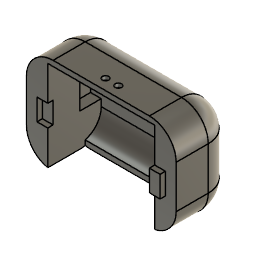
part - head front (Autodesk Fusion 360 design; units mm, degrees)
Autodesk Fusion 360 part; units mm, degrees
note: some values were not read from the file. Set by a fixed rule: which sketch regions a step uses.
sketch "Sketch6" plane through (0, 0, 0) normal (1, 0, 0) x (0, 1, 0)
  line L0 (30, 45) -> (-30, 45)
  line L1 (-55, 20) -> (-55, -20)
  line L2 (-30, -45) -> (30, -45)
  line L3 (55, -20) -> (55, 20)
  line L4 (55, 45) -> (-55, -45) construction
  line L5 (-55, 45) -> (55, -45) construction
  arc A0 (-55, -20) -> (-30, -45) centre (-30, -20) ccw
  arc A1 (55, 20) -> (30, 45) centre (30, 20) ccw
  arc A2 (-30, 45) -> (-55, 20) centre (-30, 20) ccw
  arc A3 (30, -45) -> (55, -20) centre (30, -20) ccw
  dimension "d55" = 110
  dimension "d56" = 90
  dimension "d57" = 25
  constraint horizontal L0
  constraint perpendicular L0 L1
  constraint parallel L0 L2
  constraint parallel L1 L3
  constraint coincident L4 origin
  constraint coincident L5 origin
  constraint coincident L4.end L1
  constraint coincident L4.end L2
  constraint tangent L1 A0
  constraint tangent L2 A0
  constraint coincident L4.start L3
  constraint coincident L4.start L0
  constraint tangent L3 A1
  constraint tangent L0 A1
  constraint equal A0 A1
  constraint coincident L5.start L1
  constraint coincident L5.start L0
  constraint tangent L1 A2
  constraint tangent L0 A2
  constraint equal A0 A2
  constraint coincident L5.end L2
  constraint coincident L5.end L3
  constraint tangent L2 A3
  constraint tangent L3 A3
  constraint equal A0 A3
  measures "d55" distance of L4.end L5.end
  measures "d56" distance of L5.start L4.end
  measures "d57" radius of A0
extrude "Extrude10" add sketch "Sketch6" along normal mid plane 140
fillet "Fillet11" radius 25 16 edges at (-70, 47.6777, 37.6777) (-70, 55, 0) (-70, 47.6777, -37.6777) (-70, 0, -45) (-70, -47.6777, -37.6777) (-70, -55, 0) (-70, -47.6777, 37.6777) (-70, 0, 45) (70, -47.6777, -37.6777) (70, 0, -45) (70, 47.6777, -37.6777) (70, 55, 0) (70, 47.6777, 37.6777) (70, 0, 45) (70, -47.6777, 37.6777) (70, -55, 0)
sketch "Sketch7" plane through (0, 0, 0) normal (1, 0, 0) x (0, 1, 0)
  arc A0 (-55, -20) -> (-30, -45) centre (-30, -20) ccw
  line L0 (-55, -20) -> (-55, 20)
  arc A1 (-30, 45) -> (-55, 20) centre (-30, 20) ccw
  line L1 (-30, 45) -> (30, 45)
  line L2 (55, 20) -> (55, -20)
  arc A2 (55, 20) -> (30, 45) centre (30, 20) ccw
  line L3 (30, -45) -> (-30, -45)
  arc A3 (30, -45) -> (55, -20) centre (30, -20) ccw
  line L4 (-50, -20) -> (-50, 20)
  arc A4 (-30, 40) -> (-50, 20) centre (-30, 20) ccw
  line L5 (-30, 40) -> (30, 40)
  arc A5 (50, 20) -> (30, 40) centre (30, 20) ccw
  line L6 (50, 20) -> (50, -20)
  arc A6 (30, -40) -> (50, -20) centre (30, -20) ccw
  line L7 (30, -40) -> (-30, -40)
  arc A7 (-50, -20) -> (-30, -40) centre (-30, -20) ccw
  dimension "d62" = -5
sketch "Sketch8" plane through (0, 0, 0) normal (0, 0, 1) x (1, 0, 0)
  arc A0 (45, -55) -> (70, -30) centre (45, -30) ccw
  line L0 (70, 30) -> (70, -30)
  arc A1 (70, 30) -> (45, 55) centre (45, 30) ccw
  line L1 (-45, -55) -> (45, -55)
  arc A2 (-45, 55) -> (-70, 30) centre (-45, 30) ccw
  line L2 (-70, -30) -> (-70, 30)
  arc A3 (-70, -30) -> (-45, -55) centre (-45, -30) ccw
  line L3 (-45, 55) -> (45, 55)
  line L4 (65, 30) -> (65, -30)
  arc A4 (45, -50) -> (65, -30) centre (45, -30) ccw
  line L5 (-45, -50) -> (45, -50)
  arc A5 (-65, -30) -> (-45, -50) centre (-45, -30) ccw
  line L6 (-65, -30) -> (-65, 30)
  arc A6 (-45, 50) -> (-65, 30) centre (-45, 30) ccw
  line L7 (-45, 50) -> (45, 50)
  arc A7 (65, 30) -> (45, 50) centre (45, 30) ccw
  line L8 (-45, -55) -> (-45, 55)
  line L9 (45, 55) -> (45, -55)
  dimension "d63" = -5
  constraint coincident L1.start A3.end
  constraint coincident A2.start L3.start
  constraint coincident A1.end L3.end
  constraint coincident A0.start L1.end
extrude "Extrude11" cut sketch "Sketch7" along normal mid plane 90 contours L4 A4 L5 A5 L6 A6 L7 A7
extrude "Extrude12" cut 1 faces at (15, -10, -45) along direction (0, 0, 1) blind 75
extrude "Extrude13" cut 1 faces at (15, 30, -41.6667) along direction (0, 1, 0) blind 5
extrude "Extrude14" cut 1 faces at (15, -30, -43.3333) along direction (0, -1, 0) blind 5
extrude "Extrude15" cut 1 faces at (-15, -31.6667, -40) along direction (0, 0, 1) blind 13
extrude "Extrude16" cut 1 faces at (-15, 31.6667, -40) along direction (0, 0, 1) blind 9
extrude "Extrude17" cut 1 faces at (-45, -10, -12.9099) along direction (-1, 0, 0) blind 5
extrude "Extrude25" cut 1 faces at (45, -10, -12.9099) along direction (1, 0, 0) blind 5
sketch "Sketch9" plane through (0, 0, 0) normal (0, 1, 0) x (1, 0, 0)
  line L0 (50, 43.9792) -> (50, 44.4949)
  arc A0 (50, 43.9792) -> (45, 44.4949) centre (45, 20) ccw
  arc A1 (70, 20) -> (50, 44.4949) centre (45, 20) ccw
  line L1 (-50, 44.4949) -> (-50, 43.9792)
  line L2 (-45, 44.4949) -> (45, 44.4949)
  arc A2 (-45, 44.4949) -> (-50, 43.9792) centre (-45, 20) ccw
  line L3 (70, 20) -> (70, -20)
  arc A3 (45, -45) -> (70, -20) centre (45, -20) ccw
  line L4 (-45, -45) -> (45, -45)
  arc A4 (-70, -20) -> (-45, -45) centre (-45, -20) ccw
  arc A5 (-50, 44.4949) -> (-70, 20) centre (-45, 20) ccw
  line L5 (-70, -20) -> (-70, 20)
sketch "Sketch10" plane through (0, 0, 45) normal (0, 0, 1) x (-1, 0, 0)
  line L0 (-45, 30) -> (-45, -30)
  line L1 (-45, -30) -> (45, -30)
  line L2 (45, -30) -> (45, 30)
  line L3 (45, 30) -> (-45, 30)
  circle A0 centre (6, -10) radius 1.6
  line L4 (45, 0) -> (-45, 0)
  circle A1 centre (-6, -10) radius 1.6
  circle A2 centre (6, 10) radius 1.6
  circle A3 centre (-6, 10) radius 1.6
  circle A4 centre (6, -10) radius 3
  circle A5 centre (-6, -10) radius 3
  circle A6 centre (6, 10) radius 3
  circle A7 centre (-6, 10) radius 3
  dimension "d94" = 3.2
  dimension "d95" = 6
  dimension "d96" = 10
  dimension "d99" = -12
  dimension "d100" = 20
  dimension "d101" = 6
  constraint concentric A0 A4
  measures "d94" diameter of A0
  measures "d95" horizontal distance of origin A0.centre
  measures "d96" distance of A0.centre L4
  measures "d101" diameter of A4
extrude "Extrude26" cut sketch "Sketch10" against normal blind 35 contours A0 | A1 | A2 | A3
extrude "Extrude27" cut sketch "Sketch10" against normal blind 3.5 contours A4 | A5 | A6 | A7
ref_plane "WorkPlane1" through (0, 0, 0) normal (0, -1, 0) x (0, 0, -1)
sketch "Sketch11" plane through (0, 0, 0) normal (0, -1, 0) x (-1, 0, 0)
  line L0 (-50, 44.4949) -> (-50, 43.9792)
  line L1 (50, 43.9792) -> (50, 44.4949)
  arc A0 (50, 43.9792) -> (45, 44.4949) centre (45, 20) ccw
  arc A1 (70, 20) -> (50, 44.4949) centre (45, 20) ccw
  line L2 (-45, 44.4949) -> (45, 44.4949)
  arc A2 (-45, 44.4949) -> (-50, 43.9792) centre (-45, 20) ccw
  arc A3 (-50, 44.4949) -> (-70, 20) centre (-45, 20) ccw
  line L3 (-70, -20) -> (-70, 20)
  arc A4 (-70, -20) -> (-45, -45) centre (-45, -20) ccw
  arc A5 (45, -45) -> (70, -20) centre (45, -20) ccw
  line L4 (70, 20) -> (70, -20)
  line L5 (45, -45) -> (-45, -45)
extrude "Extrude28" cut sketch "Sketch11" along normal blind 75
sketch "Sketch12" plane through (0, 0, 0) normal (0, -1, 0) x (1, 0, 0)
  line L0 (-50, -44.4949) -> (-50, 40)
  line L1 (-50, 40) -> (50, 40)
  line L2 (50, 40) -> (50, -44.4949)
  arc A0 (50, -44.4949) -> (70, -20) centre (45, -20) ccw
  line L3 (70, -20) -> (70, 20)
  arc A1 (70, 20) -> (45, 45) centre (45, 20) ccw
  line L4 (45, 45) -> (-45, 45)
  arc A2 (-45, 45) -> (-70, 20) centre (-45, 20) ccw
  line L5 (-70, 20) -> (-70, -20)
  arc A3 (-70, -20) -> (-50, -44.4949) centre (-45, -20) ccw
  line L6 (-60, 7.7526) -> (-40, 7.7526)
  line L7 (-40, 7.7526) -> (-40, -12.2474)
  line L8 (-40, -12.2474) -> (-60, -12.2474)
  line L9 (-60, -12.2474) -> (-60, 7.7526)
  line L10 (-60, 7.7526) -> (-40, -12.2474) construction
  line L11 (-40, 7.7526) -> (-60, -12.2474) construction
  line L12 (0, -53.5021) -> (0, 53.5021)
  line L13 (60, -12.2474) -> (60, 7.7526)
  line L14 (60, 7.7526) -> (40, 7.7526)
  line L15 (40, 7.7526) -> (40, -12.2474)
  line L16 (40, -12.2474) -> (60, -12.2474)
  point P0 (-50, -2.2474)
  dimension "d108" = 10
  dimension "d109" = 20
  constraint horizontal L6
  constraint perpendicular L6 L7
  constraint parallel L6 L8
  constraint parallel L7 L9
  constraint coincident L10 P0
  constraint coincident L11 P0
  constraint midpoint L0 P0
  constraint midpoint L12 origin
  constraint perpendicular L4 L12
  constraint symmetric L6.start L12 L13.end
  constraint symmetric L6.end L12 L14.end
  constraint symmetric L7.end L12 L15.end
  constraint symmetric L8.end L12 L13.start
  measures "d108" distance of L0 L9
  measures "d109" distance of L6.start L8.end
extrude "Extrude29" cut sketch "Sketch12" against normal blind 5 contours L0 L6 L8 L9
extrude "Extrude30" add sketch "Sketch12" along normal blind 5 contours L2 L13 L14 L16
sketch "Sketch15" plane through (-50, 0, 0) normal (1, 0, 0) x (0, 1, 0)
  line L0 (5, -12.2474) -> (0, -12.2474)
  line L1 (0, -12.2474) -> (0, -44.4949)
  line L2 (0, -44.4949) -> (30, -44.4949)
  arc A0 (30, -44.4949) -> (35, -43.9792) centre (30, -20) ccw
  line L3 (35, -43.9792) -> (35, -39.3649)
  arc A1 (35, -39.3649) -> (50, -20) centre (30, -20) ccw
  line L4 (50, -20) -> (50, 20)
  arc A2 (50, 20) -> (30, 40) centre (30, 20) ccw
  line L5 (30, 40) -> (0, 40)
  line L6 (0, 40) -> (0, 7.7526)
  line L7 (0, 7.7526) -> (5, 7.7526)
  line L8 (5, 7.7526) -> (5, -12.2474)
  line L9 (50, 20) -> (30, 20)
  line L10 (30, 20) -> (30, -20)
  line L11 (30, -20) -> (50, -20)
  line L12 (50, -20) -> (50, 20)
  constraint horizontal L9
  constraint vertical L10
  constraint horizontal L11
  constraint vertical L12
  constraint coincident A0.centre A1.centre
  constraint coincident L4.end A2.start
extrude "Extrude32" cut sketch "Sketch15" against normal blind 10 contours L4 L9 L10 L11 L12
sketch "Sketch13" plane through (0, 50, 0) normal (0, -1, 0) x (1, 0, 0)
  line L0 (50, 20) -> (-50, 20)
  line L1 (-50, -20) -> (50, -20)
  line L2 (50, -20) -> (50, 20)
  circle A0 centre (-29, 0) radius 4.5
  circle A1 centre (29, 0) radius 4.5
  line L3 (-59.5, 13.75) -> (-17, 13.75)
  line L4 (-17, 13.75) -> (-17, -13.75)
  line L5 (-17, -13.75) -> (-59.5, -13.75)
  line L6 (-59.5, -13.75) -> (-59.5, 13.75)
  line L7 (-50, 20) -> (-60, 20)
  line L8 (-60, 20) -> (-60, -20)
  line L9 (-60, -20) -> (-50, -20)
  dimension "d115" = 9
  dimension "d118" = 58
  dimension "d119" = 0
  dimension "d123" = 13.75
  dimension "d124" = 20
  dimension "d126" = 42.5
  dimension "d127" = 27.5
  dimension "d130" = 12
  dimension "d131" = 29
  constraint horizontal L3
  constraint vertical L4
  constraint horizontal L5
  constraint vertical L6
  measures "d115" diameter of A0
  measures "d123" distance of A0.centre L3
  measures "d124" distance of L0 A0.centre
  measures "d126" distance of L4 L6
  measures "d127" distance of L3.start L5.end
  measures "d130" distance of A0.centre L4
  measures "d131" distance of origin A0.centre
extrude "Extrude31" cut sketch "Sketch13" against normal blind 10 contours A0 | A1
chamfer "Chamfer1" distance 2 angle 45 2 edges at (24.8045, 55, -1.6273) (-33.1955, 55, -1.6273)
extrude "Extrude33" add 1 faces at (-53.3333, 36.6667, -20) along direction (0, 0, 1) blind 6.5
equation "d118 = ( 29 * 2 ) * 1 mm"
equation "d123 = ( 27.5 / 2 ) * 1 mm"
